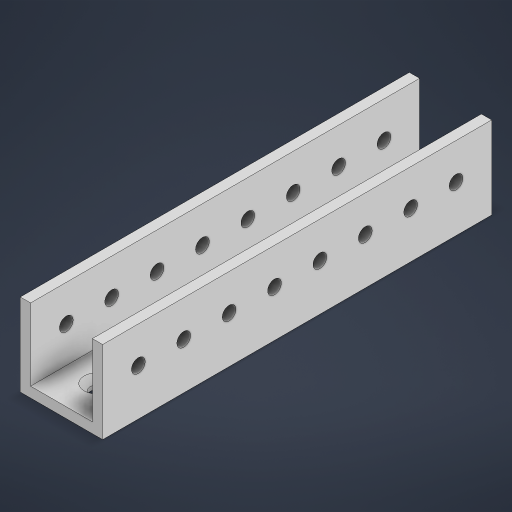
# Autodesk Inventor part: C-Channel_ArmSupport
Saved by Autodesk Inventor 2024 (Build 280153000, 153)
## iProperties
Created: 2024-01-05
Part Number: C-Channel_ArmSupport
Material: Generic
Document SubType Name: Modeling
Designer: avsar
Density: 1 g/cm^3
Appearance: Default
Author: avsar
Autodesk Inventor part; units mm, degrees
ref_plane "YZ Plane" through (0, 0, 0) normal (1, 0, 0) x (0, 1, 0)
ref_plane "XZ Plane" through (0, 0, 0) normal (0, 1, 0) x (-1, 0, 0)
ref_plane "XY Plane" through (0, 0, 0) normal (0, 0, 1) x (1, 0, 0)
sketch "Sketch1" plane through (0, 0, 0) normal (0, 0, 1) x (1, 0, 0)
  line L0 (-12.7, 0) -> (12.7, 0)
  line L1 (-12.7, 0) -> (-12.7, 25.4)
  line L2 (12.7, 0) -> (12.7, 25.4)
  line L3 (-9.525, 25.4) -> (-9.525, 3.175)
  line L4 (-9.525, 3.175) -> (9.525, 3.175)
  line L5 (9.525, 3.175) -> (9.525, 25.4)
  line L6 (-12.7, 25.4) -> (-9.525, 25.4)
  line L7 (9.525, 25.4) -> (12.7, 25.4)
  point P0 (0, 0)
  point P1 (0, 0)
  dimension "d0" = 25.4
  dimension "d1" = 25.4
  dimension "d2" = 25.4
  dimension "d3" = 3.175
  constraints: 16 end point, 2 horizontal, 2 vertical, 1 coincident, 1 collinear, 1 midpoint, 2 other
  measures "d0" distance of L0.start L0.end
  measures "d1" distance of L0.start L1.end
  measures "d2" distance of L0.end L2.end
  measures "d3" distance between parallel lines of L1 L3
extrude "Extrusion1" add sketch "Sketch1" along normal blind 120
sketch "Sketch2" plane through (-9.525, 3.175, 0) normal (0, 1, 0) x (1, 0, 0)
  circle A0 centre (9.525, -11) radius 2.1
  line L0 (-3.175, 0) -> (-3.175, -120) construction
  circle A1 centre (9.525, -25) radius 2.1
  circle A2 centre (9.525, -39) radius 2.1
  circle A3 centre (9.525, -53) radius 2.1
  circle A4 centre (9.525, -67) radius 2.1
  circle A5 centre (9.525, -81) radius 2.1
  circle A6 centre (9.525, -95) radius 2.1
  circle A7 centre (9.525, -109) radius 2.1
  line L1 (9.525, -67) -> (9.525, -53) construction
  line L2 (19.05, 0) -> (19.05, -120) projected
  line L3 (19.05, 0) -> (0, 0) projected
  point P0 (9.525, 0)
  point P1 (9.525, -60)
  point P2 (19.05, -60)
  point P3 (9.525, 0)
  dimension "d6" = 4.2
  dimension "d10" = 14
  constraints: 8 centre point, 3 midpoint, 2 end point, 2 vertical, 1 horizontal alignment, 1 vertical alignment, 14 other
  measures "d6" diameter of A0
  measures "d10" distance of A0.centre A1.centre
extrude "Extrusion2" cut sketch "Sketch2" against normal through all
sketch "Sketch3" plane through (12.7, 0, 0) normal (1, 0, 0) x (0, 0, -1)
  circle A0 centre (-11, 14.2875) radius 2.1
  line L0 (0, 3.175) -> (0, 25.4) construction
  line L1 (0, 25.4) -> (-120, 25.4) construction
  circle A1 centre (-25, 14.2875) radius 2.1
  circle A2 centre (-39, 14.2875) radius 2.1
  circle A3 centre (-53, 14.2875) radius 2.1
  circle A4 centre (-67, 14.2875) radius 2.1
  circle A5 centre (-81, 14.2875) radius 2.1
  circle A6 centre (-95, 14.2875) radius 2.1
  circle A7 centre (-109, 14.2875) radius 2.1
  line L2 (-67, 14.2875) -> (-53, 14.2875) construction
  point P0 (0, 0)
  point P1 (0, 14.2875)
  point P2 (-60, 14.2875)
  point P3 (-60, 25.4)
  dimension "d17" = 4.2
  dimension "d21" = 14
  constraints: 8 centre point, 3 midpoint, 2 end point, 2 horizontal, 1 horizontal alignment, 1 vertical alignment, 14 other
  measures "d17" diameter of A0
  measures "d21" distance of A0.centre A1.centre
extrude "Extrusion3" cut sketch "Sketch3" against normal through all
hole "Hole1" at (0, 3.175, 109) at (0, 3.175, 95) at (0, 3.175, 81) at (0, 3.175, 67) at (0, 3.175, 53) at (0, 3.175, 39) at (0, 3.175, 25) at (0, 3.175, 11) direction (0, -1, 0) diameter 4.2 end through all countersink diameter 8 countersink angle 90
body "Solid1"
